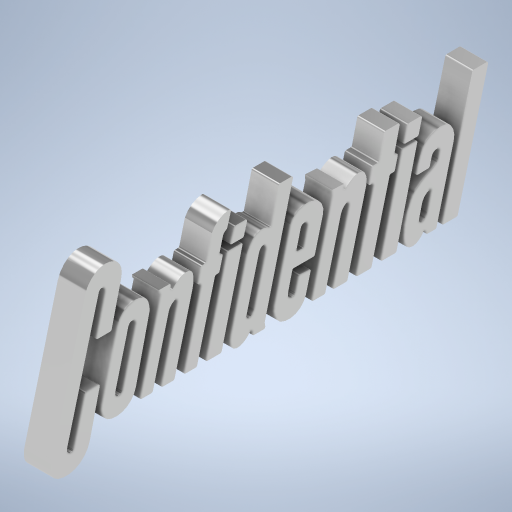
# Autodesk Inventor part: Confidential
Saved by Autodesk Inventor 2024 (Build 280153000, 153)
## iProperties
Created: 2024-08-29
Part Number: Confidential
Material: Aluminio 6061-AHC
Document SubType Name: Modeling
Designer: aless
Density: 2.7 g/cm^3
Appearance: Anodizado - Negro
Author: aless
Autodesk Inventor part; units mm, degrees
ref_plane "XZ Plane" through (0, 0, 0) normal (0, 1, 0) x (-1, 0, 0)
sketch "Boceto1" plane through (0, 0, 0) normal (1, 0, 0) x (0, 1, 0)
  line L0 (117.8279, 127.497) -> (117.8279, -120.4458) construction
  line L1 (117.8279, -120.4458) -> (0, -120.4458) construction
  line L2 (0, -120.4458) -> (0, 127.497) construction
  line L3 (0, 127.497) -> (117.8279, 127.497) construction
  line L4 (27.8242, 86.8784) -> (75.1401, 74.555)
  arc A0 (80.8863, 70.2038) -> (75.1401, 74.555) centre (72.7701, 65.4554) ccw
  arc A1 (81.0289, 63.5257) -> (80.8863, 70.2038) centre (74.9602, 66.7367) ccw
  arc A2 (76.2145, 60.6263) -> (81.0289, 63.5257) centre (76.2147, 66.0729) ccw
  arc A3 (73.6187, 60.9108) -> (76.2145, 60.6263) centre (76.2149, 72.6151) ccw
  line L5 (73.6187, 60.9108) -> (59.1706, 64.3833)
  line L6 (58.684, 65.0008) -> (58.684, 69.6552)
  line L7 (59.4758, 70.2706) -> (72.7701, 66.8832)
  arc A4 (72.7701, 66.8832) -> (74.3625, 67.4863) centre (73.1363, 68.3202) ccw
  arc A5 (74.3625, 67.4863) -> (73.7483, 69.2112) centre (73.4246, 68.1241) ccw
  line L8 (73.7483, 69.2112) -> (28.6372, 81.2187)
  arc A6 (28.6372, 81.2187) -> (26.727, 80.3786) centre (28.2075, 79.6041) ccw
  arc A7 (26.727, 80.3786) -> (26.8877, 79.0662) centre (27.7587, 79.8389) ccw
  arc A8 (26.8877, 79.0662) -> (27.2069, 78.8136) centre (27.7587, 79.8389) ccw
  line L9 (27.2069, 78.8136) -> (43.0886, 74.5863)
  line L10 (43.5602, 73.9831) -> (43.6344, 69.4946)
  line L11 (42.8531, 68.8662) -> (27.0362, 72.6151)
  arc A9 (21.5918, 76.1844) -> (27.0362, 72.6151) centre (29.2402, 81.914) ccw
  arc A10 (20.4435, 84.6322) -> (21.5918, 76.1844) centre (28.6074, 81.4399) ccw
  arc A11 (24.0007, 87.2978) -> (20.4435, 84.6322) centre (24.3719, 83.0961) ccw
  arc A12 (27.8242, 86.8784) -> (24.0007, 87.2978) centre (24.8638, 77.5291) ccw
  line L12 (36.9236, 68.1241) -> (59.2153, 62.3183)
  arc A13 (64.3169, 56.7403) -> (59.2153, 62.3183) centre (57.4642, 55.5948) ccw
  arc A14 (63.7558, 52.7386) -> (64.3169, 56.7403) centre (57.6792, 55.6308) ccw
  arc A15 (61.3735, 50.6081) -> (63.7558, 52.7386) centre (60.0233, 54.5151) ccw
  arc A16 (57.9044, 50.1175) -> (61.3735, 50.6081) centre (58.3787, 59.2741) ccw
  line L13 (57.9044, 50.1175) -> (35.8258, 55.2456)
  arc A17 (29.9931, 64.322) -> (35.8258, 55.2456) centre (37.5764, 62.7828) ccw
  arc A18 (33.893, 68.3202) -> (29.9931, 64.322) centre (35.0435, 63.2969) ccw
  arc A19 (36.1941, 68.3202) -> (33.893, 68.3202) centre (35.0435, 63.2969) ccw
  line L14 (36.1941, 68.3202) -> (36.9236, 68.1241)
  line L15 (37.9049, 63.0641) -> (57.1348, 58.0543)
  arc A20 (58.181, 56.7403) -> (57.1348, 58.0543) centre (56.7819, 56.6997) ccw
  arc A21 (56.7819, 55.3) -> (58.181, 56.7403) centre (56.7819, 56.6997) ccw
  line L16 (56.7819, 55.3) -> (37.4307, 60.2838)
  arc A22 (36.1941, 61.6966) -> (37.4307, 60.2838) centre (37.8455, 61.8945) ccw
  arc A23 (37.9049, 63.0641) -> (36.1941, 61.6966) centre (37.4735, 61.8499) ccw
  line L17 (31.3113, 48.8406) -> (54.1555, 42.8909)
  arc A24 (56.7819, 40.7835) -> (54.1555, 42.8909) centre (53.118, 38.9078) ccw
  arc A25 (56.7819, 40.0187) -> (56.7819, 40.7835) centre (56.0349, 40.4011) ccw
  arc A26 (56.2905, 39.6018) -> (56.7819, 40.0187) centre (56.0349, 40.4011) ccw
  arc A27 (55.7794, 39.6018) -> (56.2905, 39.6018) centre (56.0349, 40.4011) ccw
  line L18 (55.7794, 39.6018) -> (31.6274, 45.727)
  line L19 (30.8363, 45.1115) -> (30.8363, 41.2743)
  line L20 (31.3113, 40.6598) -> (57.3535, 33.8771)
  arc A28 (57.3535, 33.8771) -> (62.0718, 33.7602) centre (59.9624, 43.894) ccw
  arc A29 (62.0718, 33.7602) -> (63.7558, 35.4689) centre (61.6307, 35.8791) ccw
  arc A30 (63.7558, 35.4689) -> (63.1723, 38.625) centre (59.4372, 36.3024) ccw
  arc A31 (63.1723, 38.625) -> (60.9152, 41.4093) centre (50.9524, 31.0261) ccw
  arc A32 (60.8406, 42.1181) -> (60.9152, 41.4093) centre (61.2976, 41.8079) ccw
  line L21 (60.8406, 42.1181) -> (62.4315, 42.1181)
  line L22 (63.0665, 42.7531) -> (63.0665, 46.6111)
  arc A33 (63.0665, 46.6111) -> (61.4644, 45.9276) centre (62.8943, 44.7952) ccw
  line L23 (61.4644, 45.9276) -> (31.6314, 53.6976)
  line L24 (30.8363, 36.5132) -> (30.8363, 32.7811)
  line L25 (31.3112, 32.1666) -> (56.8786, 25.5047)
  line L26 (57.3535, 24.8902) -> (57.3535, 24.3295)
  line L27 (57.8284, 23.715) -> (62.2713, 22.5574)
  line L28 (63.0665, 23.1719) -> (63.0665, 23.0707)
  line L29 (63.8616, 23.6852) -> (68.9851, 22.3502)
  arc A34 (70.142, 21.1532) -> (68.9851, 22.3502) centre (67.7077, 19.9581) ccw
  arc A35 (76.0914, 20.0813) -> (71.714, 26.6325) centre (68.4116, 19.6878) ccw
  line L30 (71.714, 26.6325) -> (63.5447, 28.7138)
  line L31 (63.0665, 29.3291) -> (63.0665, 30.2732)
  line L32 (62.5789, 30.8909) -> (58.1359, 31.9512)
  line L33 (57.3535, 31.3335) -> (57.3535, 31.3917)
  line L34 (56.5617, 30.7764) -> (31.6281, 37.1286)
  line L35 (62.873, 20.4416) -> (62.873, 15.6867)
  line L36 (62.0812, 15.0714) -> (31.3146, 22.9096)
  line L37 (30.8363, 23.5249) -> (30.8363, 28.2798)
  line L38 (31.6281, 28.8951) -> (62.3948, 21.0569)
  line L39 (64.3438, 19.1211) -> (64.3438, 15.1264)
  line L40 (64.8061, 14.5153) -> (68.9407, 13.3464)
  line L41 (69.7485, 13.9574) -> (69.7485, 17.7173)
  line L42 (69.3176, 18.3186) -> (65.183, 19.7224)
  line L43 (36.669, 19.0898) -> (57.1106, 13.882)
  arc A36 (62.1786, 11.1511) -> (57.1106, 13.882) centre (54.1783, 2.3725) ccw
  arc A37 (62.873, 5.2846) -> (62.1786, 11.1511) centre (59.1402, 7.8171) ccw
  arc A38 (62.873, 5.2846) -> (62.7789, 4.4125) centre (63.6461, 4.7601) ccw
  line L44 (62.7789, 4.4125) -> (74.6554, 1.5184)
  line L45 (75.1401, 0.9014) -> (75.1401, -3.3031)
  line L46 (74.3483, -3.9184) -> (32.6153, 6.715)
  line L47 (32.6153, 6.715) -> (31.2476, 6.5045)
  line L48 (30.516, 7.1321) -> (30.516, 10.7623)
  line L49 (31.151, 11.3973) -> (32.1388, 11.3973)
  arc A39 (32.1388, 11.3973) -> (32.4131, 12.1287) centre (32.1388, 11.8144) ccw
  arc A40 (31.3274, 13.118) -> (32.4131, 12.1287) centre (54.9112, 37.9078) ccw
  arc A41 (29.5356, 16.0569) -> (31.3274, 13.118) centre (35.8937, 17.9178) ccw
  arc A42 (31.8649, 19.6878) -> (29.5356, 16.0569) centre (32.2787, 16.8597) ccw
  arc A43 (34.4434, 19.6568) -> (31.8649, 19.6878) centre (33.0562, 11.5457) ccw
  line L50 (34.4434, 19.6568) -> (36.669, 19.0898)
  line L51 (38.869, 13.4398) -> (56.2905, 8.8946)
  arc A44 (57.81, 8.0154) -> (56.2905, 8.8946) centre (55.4577, 5.7025) ccw
  arc A45 (57.81, 6.715) -> (57.81, 8.0154) centre (57.1487, 7.3652) ccw
  arc A46 (56.1069, 6.2649) -> (57.81, 6.715) centre (56.579, 7.9254) ccw
  line L52 (56.1069, 6.2649) -> (39.5095, 10.5876)
  arc A47 (37.2122, 11.9929) -> (39.5095, 10.5876) centre (40.6798, 15.0813) ccw
  arc A48 (37.9049, 13.5995) -> (37.2122, 11.9929) centre (37.9216, 12.6397) ccw
  arc A49 (38.869, 13.4398) -> (37.9049, 13.5995) centre (37.9216, 10.7111) ccw
  line L53 (45.3223, -12.2295) -> (57.1649, -15.3085)
  arc A50 (57.1649, -15.3085) -> (62.9646, -12.3304) centre (58.1292, -10.0501) ccw
  arc A51 (62.9646, -12.3304) -> (62.9081, -5.7311) centre (56.0917, -9.0893) ccw
  arc A52 (62.9081, -5.7311) -> (59.8125, -2.9091) centre (57.1469, -8.942) ccw
  line L54 (59.8125, -2.9091) -> (36.3261, 3.1529)
  arc A53 (36.3261, 3.1529) -> (29.8726, 0.859) centre (34.7972, -2.7707) ccw
  arc A54 (29.8726, 0.859) -> (33.893, -8.8212) centre (35.8124, -2.3491) ccw
  line L55 (33.893, -8.8212) -> (40.6779, -10.5883)
  line L56 (41.4717, -10.0136) -> (41.6849, -6.614)
  line L57 (41.2098, -5.9594) -> (36.669, -4.7878)
  line L58 (30.516, -11.6026) -> (30.516, -15.5402)
  line L59 (30.991, -16.1547) -> (53.6764, -22.0621)
  arc A55 (56.0917, -23.8418) -> (53.6764, -22.0621) centre (52.4087, -26.3113) ccw
  arc A56 (55.9263, -24.8577) -> (56.0917, -23.8418) centre (55.466, -24.2613) ccw
  arc A57 (54.7861, -25.0602) -> (55.9263, -24.8577) centre (55.1625, -23.8681) ccw
  line L60 (54.7861, -25.0602) -> (31.272, -18.9338)
  line L61 (30.4769, -19.5483) -> (30.4769, -23.8909)
  line L62 (30.9527, -24.5056) -> (58.2199, -31.5691)
  arc A58 (58.2199, -31.5691) -> (62.5911, -31.0129) centre (59.7093, -25.8194) ccw
  arc A59 (62.5911, -31.0129) -> (63.6759, -29.5252) centre (61.5292, -29.0992) ccw
  arc A60 (63.6759, -29.5252) -> (63.2975, -26.8002) centre (59.5586, -28.7081) ccw
  arc A61 (63.2975, -26.8002) -> (60.9548, -23.5494) centre (51.5587, -32.7903) ccw
  arc A62 (61.1049, -23.0402) -> (60.9548, -23.5494) centre (61.1712, -23.3365) ccw
  line L63 (61.1049, -23.0402) -> (62.873, -23.15)
  line L64 (62.873, -23.15) -> (63.1476, -18.7267)
  arc A63 (63.1476, -18.7267) -> (61.4325, -18.7786) centre (62.3704, -21.4038) ccw
  line L65 (61.4325, -18.7786) -> (31.31, -10.9879)
  line L66 (30.2373, -28.3064) -> (30.2373, -32.9608)
  line L67 (30.7133, -33.5756) -> (56.8775, -40.3426)
  line L68 (57.3535, -40.9574) -> (57.3535, -41.7743)
  line L69 (57.8291, -42.3889) -> (61.9845, -43.4664)
  line L70 (62.7789, -42.8517) -> (62.7789, -42.873)
  line L71 (63.5608, -42.2552) -> (71.5806, -44.1617)
  line L72 (72.3624, -43.5439) -> (72.3624, -38.9039)
  line L73 (71.8758, -38.2865) -> (63.8571, -36.3592)
  line L74 (63.3705, -35.7418) -> (63.3705, -34.1705)
  line L75 (62.8839, -33.5531) -> (58.3952, -32.4742)
  line L76 (57.6118, -33.0916) -> (57.6118, -33.6252)
  line L77 (56.8205, -34.2407) -> (31.0286, -27.6909)
  line L78 (50.4422, -5.302) -> (56.5664, -6.8717)
  arc A64 (57.4515, -7.449) -> (56.5664, -6.8717) centre (56.1581, -8.4647) ccw
  arc A65 (57.3339, -9.1476) -> (57.4515, -7.449) centre (56.4528, -8.2333) ccw
  arc A66 (56.2106, -9.4797) -> (57.3339, -9.1476) centre (56.4528, -8.2333) ccw
  line L79 (56.2106, -9.4797) -> (50.117, -7.9658)
  arc A67 (49.718, -7.6122) -> (50.117, -7.9658) centre (50.2558, -7.4072) ccw
  line L80 (49.718, -7.6122) -> (49.718, -5.4964)
  arc A68 (50.4422, -5.302) -> (49.718, -5.4964) centre (50.2254, -5.9407) ccw
  line L81 (30.6265, -37.6121) -> (30.6265, -42.3741)
  line L82 (31.1086, -42.9904) -> (62.5924, -50.7976)
  line L83 (63.3803, -50.1812) -> (63.3803, -45.4192)
  line L84 (62.8981, -44.8029) -> (31.4143, -36.9957)
  line L85 (64.4911, -46.2402) -> (64.4911, -50.7586)
  line L86 (64.9719, -51.3746) -> (69.7099, -52.5607)
  line L87 (70.4991, -51.9447) -> (70.4991, -47.4263)
  line L88 (70.0183, -46.8103) -> (65.2803, -45.6242)
  line L89 (51.9472, -50.9917) -> (52.037, -54.9166)
  line L90 (52.5107, -55.5163) -> (55.1625, -56.2117)
  arc A69 (56.8128, -58.5311) -> (55.1625, -56.2117) centre (54.9058, -58.1412) ccw
  arc A70 (56.6362, -58.8812) -> (56.8128, -58.5311) centre (56.0808, -58.3814) ccw
  arc A71 (55.8556, -59.2079) -> (56.6362, -58.8812) centre (55.9004, -58.219) ccw
  line L91 (55.8556, -59.2079) -> (53.6764, -58.7179)
  arc A72 (52.4087, -57.953) -> (53.6764, -58.7179) centre (54.19, -56.4338) ccw
  arc A73 (50.8164, -55.3949) -> (52.4087, -57.953) centre (60.1096, -51.385) ccw
  arc A74 (50.8164, -55.3949) -> (47.6005, -50.2227) centre (31.9696, -63.5271) ccw
  arc A75 (47.6005, -50.2227) -> (45.1488, -48.3404) centre (41.9786, -55.0079) ccw
  arc A76 (45.1488, -48.3404) -> (34.4434, -45.6426) centre (34.4119, -68.3567) ccw
  arc A77 (34.4434, -45.6426) -> (31.8649, -46.0052) centre (34.4306, -54.9001) ccw
  arc A78 (31.8649, -46.0052) -> (29.8566, -50.4055) centre (32.748, -49.0667) ccw
  arc A79 (29.8566, -50.4055) -> (32.2787, -53.0619) centre (35.2768, -47.8959) ccw
  arc A80 (32.2787, -53.797) -> (32.2787, -53.0619) centre (32.0654, -53.4295) ccw
  line L92 (32.2787, -53.797) -> (31.3077, -54.1022)
  line L93 (30.8631, -54.708) -> (30.8631, -57.4617)
  line L94 (31.3386, -58.0764) -> (56.2826, -64.5465)
  arc A81 (56.2826, -64.5465) -> (61.9889, -63.3288) centre (57.9192, -58.2368) ccw
  arc A82 (61.9889, -63.3288) -> (63.1723, -61.5039) centre (59.8387, -60.6384) ccw
  arc A83 (63.1723, -61.5039) -> (59.8387, -52.6888) centre (55.2733, -59.4532) ccw
  arc A84 (59.8387, -52.6888) -> (52.6967, -50.3526) centre (47.6341, -77.9138) ccw
  line L95 (38.3938, -54.62) -> (44.5323, -56.0975)
  arc A85 (44.5323, -56.0975) -> (44.9856, -55.8033) centre (44.6194, -55.7355) ccw
  arc A86 (44.9856, -55.8033) -> (42.1056, -52.6888) centre (40.8142, -56.7718) ccw
  line L96 (42.1056, -52.6888) -> (36.9236, -51.385)
  arc A87 (36.9236, -51.385) -> (35.8045, -52.6888) centre (36.8051, -52.4155) ccw
  arc A88 (35.8045, -52.6888) -> (38.3938, -54.62) centre (39.1529, -50.9007) ccw
  line L97 (30.9048, -60.6954) -> (30.9048, -65.4578)
  line L98 (31.3789, -66.0721) -> (74.9664, -77.4901)
  line L99 (75.7623, -76.8706) -> (75.7235, -72.0981)
  line L100 (75.2494, -71.4889) -> (31.7007, -60.0811)
  arc A89 (59.4758, 70.2706) -> (58.684, 69.6552) centre (59.319, 69.6552) ccw
  arc A90 (58.684, 65.0008) -> (59.1706, 64.3833) centre (59.319, 65.0008) ccw
  arc A91 (43.5602, 73.9831) -> (43.0886, 74.5863) centre (42.9253, 73.9726) ccw
  arc A92 (42.8531, 68.8662) -> (43.6344, 69.4946) centre (42.9995, 69.4841) ccw
  line L101 (30.8363, 49.4551) -> (30.8363, 53.0831)
  arc A93 (31.6314, 53.6976) -> (30.8363, 53.0831) centre (31.4713, 53.0831) ccw
  arc A94 (30.8363, 49.4551) -> (31.3113, 48.8406) centre (31.4713, 49.4551) ccw
  arc A95 (30.8363, 41.2743) -> (31.3113, 40.6598) centre (31.4713, 41.2743) ccw
  arc A96 (62.4315, 42.1181) -> (63.0665, 42.7531) centre (62.4315, 42.7531) ccw
  arc A97 (31.6274, 45.727) -> (30.8363, 45.1115) centre (31.4713, 45.1115) ccw
  arc A98 (31.6281, 37.1286) -> (30.8363, 36.5132) centre (31.4713, 36.5132) ccw
  arc A99 (30.8363, 32.7811) -> (31.3112, 32.1666) centre (31.4713, 32.7811) ccw
  arc A100 (31.6281, 28.8951) -> (30.8363, 28.2798) centre (31.4713, 28.2798) ccw
  arc A101 (30.8363, 23.5249) -> (31.3146, 22.9096) centre (31.4713, 23.5249) ccw
  arc A102 (56.5617, 30.7764) -> (57.3535, 31.3917) centre (56.7185, 31.3917) ccw
  arc A103 (58.1359, 31.9512) -> (57.3535, 31.3335) centre (57.9885, 31.3335) ccw
  arc A104 (63.0665, 30.2732) -> (62.5789, 30.8909) centre (62.4315, 30.2732) ccw
  arc A105 (63.0665, 29.3291) -> (63.5447, 28.7138) centre (63.7015, 29.3291) ccw
  line L102 (75.2794, 19.4392) -> (70.5342, 20.8234)
  arc A106 (70.142, 21.1532) -> (70.5342, 20.8234) centre (70.712, 21.433) ccw
  arc A107 (75.2794, 19.4392) -> (76.0914, 20.0813) centre (75.4573, 20.0488) ccw
  arc A108 (63.8616, 23.6852) -> (63.0665, 23.0707) centre (63.7015, 23.0707) ccw
  arc A109 (62.2713, 22.5574) -> (63.0665, 23.1719) centre (62.4315, 23.1719) ccw
  arc A110 (57.3535, 24.3295) -> (57.8284, 23.715) centre (57.9885, 24.3295) ccw
  arc A111 (57.3535, 24.8902) -> (56.8786, 25.5047) centre (56.7185, 24.8902) ccw
  arc A112 (62.873, 20.4416) -> (62.3948, 21.0569) centre (62.238, 20.4416) ccw
  arc A113 (62.0812, 15.0714) -> (62.873, 15.6867) centre (62.238, 15.6867) ccw
  arc A114 (65.183, 19.7224) -> (64.3438, 19.1211) centre (64.9788, 19.1211) ccw
  arc A115 (64.3438, 15.1264) -> (64.8061, 14.5153) centre (64.9788, 15.1264) ccw
  arc A116 (68.9407, 13.3464) -> (69.7485, 13.9574) centre (69.1135, 13.9574) ccw
  arc A117 (69.7485, 17.7173) -> (69.3176, 18.3186) centre (69.1135, 17.7173) ccw
  arc A118 (75.1401, 0.9014) -> (74.6554, 1.5184) centre (74.5051, 0.9014) ccw
  arc A119 (74.3483, -3.9184) -> (75.1401, -3.3031) centre (74.5051, -3.3031) ccw
  arc A120 (30.516, 7.1321) -> (31.2476, 6.5045) centre (31.151, 7.1321) ccw
  arc A121 (31.151, 11.3973) -> (30.516, 10.7623) centre (31.151, 10.7623) ccw
  arc A122 (41.6849, -6.614) -> (41.2098, -5.9594) centre (41.0511, -6.5742) ccw
  arc A123 (40.6779, -10.5883) -> (41.4717, -10.0136) centre (40.8379, -9.9738) ccw
  arc A124 (36.594, -2.1105) -> (36.669, -4.7878) centre (37.1351, -3.4351) ccw
  arc A125 (38.2113, -2.1672) -> (36.594, -2.1105) centre (37.2938, -5.2432) ccw
  line L103 (38.2113, -2.1672) -> (44.3642, -3.6853)
  line L104 (44.8471, -4.3018) -> (44.8471, -11.6149)
  arc A126 (44.8471, -4.3018) -> (44.3642, -3.6853) centre (44.2121, -4.3018) ccw
  arc A127 (44.8471, -11.6149) -> (45.3223, -12.2295) centre (45.4821, -11.6149) ccw
  arc A128 (31.31, -10.9879) -> (30.516, -11.6026) centre (31.151, -11.6026) ccw
  arc A129 (30.516, -15.5402) -> (30.991, -16.1547) centre (31.151, -15.5402) ccw
  arc A130 (30.4769, -23.8909) -> (30.9527, -24.5056) centre (31.1119, -23.8909) ccw
  arc A131 (31.272, -18.9338) -> (30.4769, -19.5483) centre (31.1119, -19.5483) ccw
  arc A132 (31.0286, -27.6909) -> (30.2373, -28.3064) centre (30.8723, -28.3064) ccw
  arc A133 (30.2373, -32.9608) -> (30.7133, -33.5756) centre (30.8723, -32.9608) ccw
  arc A134 (57.3535, -40.9574) -> (56.8775, -40.3426) centre (56.7185, -40.9574) ccw
  arc A135 (57.3535, -41.7743) -> (57.8291, -42.3889) centre (57.9885, -41.7743) ccw
  arc A136 (61.9845, -43.4664) -> (62.7789, -42.8517) centre (62.1439, -42.8517) ccw
  arc A137 (63.5608, -42.2552) -> (62.7789, -42.873) centre (63.4139, -42.873) ccw
  arc A138 (71.5806, -44.1617) -> (72.3624, -43.5439) centre (71.7274, -43.5439) ccw
  arc A139 (72.3624, -38.9039) -> (71.8758, -38.2865) centre (71.7274, -38.9039) ccw
  arc A140 (63.3705, -35.7418) -> (63.8571, -36.3592) centre (64.0055, -35.7418) ccw
  arc A141 (63.3705, -34.1705) -> (62.8839, -33.5531) centre (62.7355, -34.1705) ccw
  arc A142 (58.3952, -32.4742) -> (57.6118, -33.0916) centre (58.2468, -33.0916) ccw
  arc A143 (56.8205, -34.2407) -> (57.6118, -33.6252) centre (56.9768, -33.6252) ccw
  arc A144 (31.4143, -36.9957) -> (30.6265, -37.6121) centre (31.2615, -37.6121) ccw
  arc A145 (30.6265, -42.3741) -> (31.1086, -42.9904) centre (31.2615, -42.3741) ccw
  arc A146 (63.3803, -45.4192) -> (62.8981, -44.8029) centre (62.7453, -45.4192) ccw
  arc A147 (62.5924, -50.7976) -> (63.3803, -50.1812) centre (62.7453, -50.1812) ccw
  arc A148 (65.2803, -45.6242) -> (64.4911, -46.2402) centre (65.1261, -46.2402) ccw
  arc A149 (64.4911, -50.7586) -> (64.9719, -51.3746) centre (65.1261, -50.7586) ccw
  arc A150 (69.7099, -52.5607) -> (70.4991, -51.9447) centre (69.8641, -51.9447) ccw
  arc A151 (70.4991, -47.4263) -> (70.0183, -46.8103) centre (69.8641, -47.4263) ccw
  arc A152 (52.6967, -50.3526) -> (51.9472, -50.9917) centre (52.582, -50.9771) ccw
  arc A153 (52.037, -54.9166) -> (52.5107, -55.5163) centre (52.6718, -54.9021) ccw
  arc A154 (31.3077, -54.1022) -> (30.8631, -54.708) centre (31.4981, -54.708) ccw
  arc A155 (30.8631, -57.4617) -> (31.3386, -58.0764) centre (31.4981, -57.4617) ccw
  arc A156 (31.7007, -60.0811) -> (30.9048, -60.6954) centre (31.5398, -60.6954) ccw
  arc A157 (30.9048, -65.4578) -> (31.3789, -66.0721) centre (31.5398, -65.4578) ccw
  arc A158 (74.9664, -77.4901) -> (75.7623, -76.8706) centre (75.1273, -76.8758) ccw
  arc A159 (75.7235, -72.0981) -> (75.2494, -71.4889) centre (75.0885, -72.1032) ccw
  point P0 (0, 0)
  point P1 (63.0665, 23.8924)
  point P2 (70.2481, 20.9068)
  point P3 (76.0863, 19.2038)
  point P4 (72.3624, -44.3476)
  point P5 (70.4991, -52.7582)
  point P6 (51.9296, -50.2227)
  dimension "d5" = 0.635
  dimension "d7" = 0.635
  dimension "d8" = 0.635
  dimension "d9" = 0.635
  dimension "d10" = 0.635
  constraints: 331 point on circle, 210 tangent, 202 end point, 160 centre point, 69 equal radius, 20 parallel, 18 vertical, 13 point on line, 3 perpendicular, 1 horizontal, 2 other
  measures "d5" radius of A89
  measures "d7" radius of A93
  measures "d8" radius of A106
  measures "d9" radius of A126
  measures "d10" radius of A132
extrude "Extrusión1" add sketch "Boceto1" along normal blind 10.16 contours L4 A0 A1 A2 A3 L5 A90 L6 A89 L7 A4 A5 L8 A6 A7 A8 L9 A91 L10 A92 L11 A9 A10 A11 A12 | L12 A13 A14 A15 A16 L13 A17 A18 A19 L14 | A94 L101 A93 L23 A33 L22 A96 L21 A32 A31 A30 A29 A28 L20 A95 L19 A97 L18 A27 A26 A25 A24 L17 | A98 L34 A102 A103 L32 A104 L31 A105 L30 A35 A107 L102 A106 A34 L29 A108 L28 A109 L27 A110 L26 A111 L25 A99 L24 | L35 A113 L36 A101 L37 A100 L38 A112 | A114 L42 A117 L41 A116 L40 A115 L39 | L43 A36 A37 A38 L44 A118 L45 A119 L46 L47 A120 L48 A121 L49 A39 A40 A41 A42 A43 L50 | L51 A44 A45 A46 L52 A47 A48 A49 | A127 L104 A126 L103 A125 A124 L57 A122 L56 A123 L55 A54 A53 L54 A52 A51 A50 L53 | A128 L65 A63 L64 L63 A62 A61 A60 A59 A58 L62 A130 L61 A131 L60 A57 A56 A55 L59 A129 L58 | A132 L77 A143 L76 A142 L75 A141 L74 A140 L73 A139 L72 A138 L71 A137 L70 A136 L69 A135 L68 A134 L67 A133 L66 | A144 L84 A146 L83 A147 L82 A145 L81 | A148 L88 A151 L87 A150 L86 A149 L85 | A152 A84 A83 A82 A81 L94 A155 L93 A154 L92 A80 A79 A78 A77 A76 A75 A74 A73 A72 L91 A71 A70 A69 L90 A153 L89 | A156 L100 A159 L99 A158 L98 A157 L97
extrude "Extrusión2" cut sketch "Boceto1" along normal blind 10.16 contours L51 A44 A45 A46 L52 A47 A48 A49
ref_plane "Plano de trabajo1" through (-2828.925, 0, 0) normal (1, 0, 0) x (0, 1, 0)
ref_plane "Plano de trabajo2" through (-790.575, 0, 0) normal (1, 0, 0) x (0, 1, 0)
